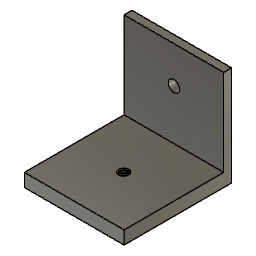
CCM_G01 side mounting plate (Autodesk Fusion 360 design; units mm, degrees)
Autodesk Fusion 360 part; units mm, degrees
box "BoxPrimitive1" add length 38.1 width 38.1 height 5 placed x (0, -1, 0) y (1, 0, 0) z (0, 0, 1) at (0, 0, 0) makes body 1
cylinder "CylinderPrimitive1" add diameter 4.166 height 5 placed x (1, 0, 0) y (0, 1, 0) z (0, 0, 1) at (0, 0, 0) separate body makes body 2
move_body "Move1" bodies 2 to x (1, 0, 0) y (0, 1, 0) z (0, 0, 1) at (19.05, -19.05, 0)
combine "Combine1" operation cut target body 1 tool bodies 2
thread "Thread1" "ANSI Unified Screw Threads 0.164(#8) 8-32 UNC 3B" major diameter 4.1656 minor diameter 3.4163 pitch 0.7937 angle 60 modelled right hand crest width 0.2414 on face at (21.1226, -19.2574, 3.3333) crest through (20.7582, -19.05, 0.1984) on bodies 1
box "BoxPrimitive3" add length 3 width 38.1 height 38.1 placed x (0, 1, 0) y (-1, 0, 0) z (0, 0, 1) at (38.1, 0, 0) separate body makes body 3
combine "Combine2" operation add target body 1 tool bodies 3
cylinder "CylinderPrimitive2" add diameter 4.3 height 3 placed x (1, 0, 0) y (0, 0, -1) z (0, 1, 0) at (0, 0, 0) separate body makes body 4
move_body "Move2" bodies 4 to x (1, 0, 0) y (0, 1, 0) z (0, 0, 1) at (19.05, 0, 24.05)
combine "Combine3" operation cut target body 1 tool bodies 4
